Autodesk Fusion 360 part; units mm, degrees
(part 5 of 5)
  spline S1328 degree 3 poles (-71.2858, -117.1443) (-71.9506, -117.9779) (-71.7606, -118.0412) (-71.0536, -117.2287) knots 0 0 0 0 1 1 1 1
  spline S1329 degree 3 poles (-71.0536, -117.2287) (-70.7054, -116.8172) (-70.3889, -116.4795) (-70.3678, -116.4795) knots 0 0 0 0 1 1 1 1
  spline S1330 degree 3 poles (-70.3678, -116.4795) (-70.3467, -116.4795) (-70.3678, -116.5956) (-70.4205, -116.7222) knots 0 0 0 0 1 1 1 1
  spline S1331 degree 3 poles (-70.4205, -116.7222) (-70.5577, -117.0704) (-70.5682, -119.7401) (-70.4416, -120.8692) knots 0 0 0 0 1 1 1 1
  spline S1332 degree 3 poles (-70.4416, -120.8692) (-70.3783, -121.3862) (-70.3044, -122.3148) (-70.2622, -122.9374) knots 0 0 0 0 1 1 1 1
  spline S1333 degree 3 poles (-70.2622, -122.9374) (-70.1778, -124.3197) (-70.315, -124.7945) (-71.1381, -125.8708) knots 0 0 0 0 1 1 1 1
  spline S1334 degree 3 poles (-71.1381, -125.8708) (-71.7606, -126.6833) (-71.8978, -127.1054) (-71.328, -126.4512) knots 0 0 0 0 1 1 1 1
  spline S1335 degree 3 poles (-71.328, -126.4512) (-70.2728, -125.2271) (-69.1543, -122.8002) (-68.8061, -120.9114) knots 0 0 0 0 1 1 1 1
  spline S1336 degree 3 poles (-68.8061, -120.9114) (-68.6056, -119.8984) (-68.6161, -119.9617) (-68.7216, -119.9617) knots 0 0 0 0 1 1 1 1
  spline S1337 degree 3 poles (-68.7216, -119.9617) (-68.7638, -119.9617) (-68.8588, -120.3205) (-68.9327, -120.7636) knots 0 0 0 0 1 1 1 1
  spline S1338 degree 3 poles (-68.9327, -120.7636) (-69.0488, -121.5445) (-69.5764, -123.2434) (-69.8613, -123.7604) knots 0 0 0 0 1 1 1 1
  spline S1339 degree 3 poles (-69.8613, -123.7604) (-69.9879, -123.9926) (-69.9984, -123.9081) (-70.009, -122.9162) knots 0 0 0 0 1 1 1 1
  spline S1340 degree 3 poles (-70.009, -122.9162) (-70.0195, -122.3042) (-70.0406, -121.6606) (-70.0723, -121.4917) knots 0 0 0 0 1 1 1 1
  spline S1341 degree 3 poles (-70.0723, -121.4917) (-70.2517, -120.2888) (-70.3044, -117.6719) (-70.1778, -116.6378) knots 0 0 0 0 1 1 1 1
  spline S1342 degree 3 poles (-70.1778, -116.6378) (-70.1251, -116.1418) (-70.0617, -116.0574) (-69.2176, -115.2344) knots 0 0 0 0 1 1 1 1
  spline S1343 degree 3 poles (-69.2176, -115.2344) (-68.2468, -114.3058) (-68.1413, -114.0842) (-69.0065, -114.8123) knots 0 0 0 0 1 1 1 1
  spline S1344 degree 3 poles (-42.4787, -115.3927) (-41.7084, -116.1313) (-41.6029, -116.2685) (-41.5185, -116.7433) knots 0 0 0 0 1 1 1 1
  spline S1345 degree 3 poles (-41.5185, -116.7433) (-41.413, -117.3026) (-41.4657, -120.9219) (-41.5818, -121.5445) knots 0 0 0 0 1 1 1 1
  spline S1346 degree 3 poles (-41.5818, -121.5445) (-41.624, -121.745) (-41.6662, -122.4203) (-41.6662, -123.0429) knots 0 0 0 0 1 1 1 1
  spline S1347 degree 3 poles (-41.6662, -123.0429) (-41.6768, -123.6654) (-41.7084, -124.1403) (-41.7401, -124.0981) knots 0 0 0 0 1 1 1 1
  spline S1348 degree 3 poles (-41.7401, -124.0981) (-41.93, -123.8976) (-42.5948, -121.861) (-42.7531, -120.9958) knots 0 0 0 0 1 1 1 1
  spline S1349 degree 3 poles (-42.7531, -120.9958) (-42.8586, -120.4576) (-42.9536, -120.12) (-42.9747, -120.2466) knots 0 0 0 0 1 1 1 1
  spline S1350 degree 3 poles (-42.9747, -120.2466) (-43.0802, -120.9747) (-42.3416, -123.3489) (-41.5502, -124.8051) knots 0 0 0 0 1 1 1 1
  spline S1351 degree 3 poles (-41.5502, -124.8051) (-41.0226, -125.8075) (-40.1256, -127.0104) (-40.0623, -126.8311) knots 0 0 0 0 1 1 1 1
  spline S1352 degree 3 poles (-40.0623, -126.8311) (-40.0412, -126.7572) (-40.1573, -126.5356) (-40.3261, -126.314) knots 0 0 0 0 1 1 1 1
  spline S1353 degree 3 poles (-40.3261, -126.314) (-40.6427, -125.8919) (-40.8326, -125.5859) (-41.2653, -124.7734) knots 0 0 0 0 1 1 1 1
  spline S1354 degree 3 poles (-41.2653, -124.7734) (-41.5185, -124.288) (-41.5291, -124.2036) (-41.4763, -123.1378) knots 0 0 0 0 1 1 1 1
  spline S1355 degree 3 poles (-41.4763, -123.1378) (-41.4446, -122.5258) (-41.3813, -121.6606) (-41.3391, -121.2279) knots 0 0 0 0 1 1 1 1
  spline S1356 degree 3 poles (-41.3391, -121.2279) (-41.2864, -120.7953) (-41.2547, -119.5924) (-41.2547, -118.5688) knots 0 0 0 0 1 1 1 1
  line L192 (-41.2547, -118.5688) -> (-41.2547, -116.7011)
  line L193 (-41.2547, -116.7011) -> (-40.9487, -116.986)
  spline S1357 degree 3 poles (-40.9487, -116.986) (-40.7799, -117.1443) (-40.5161, -117.4609) (-40.3472, -117.6824) knots 0 0 0 0 1 1 1 1
  spline S1358 degree 3 poles (-40.3472, -117.6824) (-40.1784, -117.904) (-40.0412, -118.0201) (-40.0412, -117.9357) knots 0 0 0 0 1 1 1 1
  spline S1359 degree 3 poles (-40.0412, -117.9357) (-40.0412, -117.6297) (-41.1386, -116.3845) (-42.4154, -115.2449) knots 0 0 0 0 1 1 1 1
  spline S1360 degree 3 poles (-42.4154, -115.2449) (-43.4601, -114.3058) (-43.5128, -114.4219) (-42.4787, -115.3927) knots 0 0 0 0 1 1 1 1
  spline S1361 degree 3 poles (-65.039, -118.3367) (-65.039, -118.4527) (-65.0073, -118.4844) (-64.9757, -118.4) knots 0 0 0 0 1 1 1 1
  spline S1362 degree 3 poles (-64.9757, -118.4) (-64.944, -118.3261) (-64.9546, -118.2311) (-64.9862, -118.1995) knots 0 0 0 0 1 1 1 1
  spline S1363 degree 3 poles (-64.9862, -118.1995) (-65.0179, -118.1573) (-65.0495, -118.2206) (-65.039, -118.3367) knots 0 0 0 0 1 1 1 1
  spline S1364 degree 3 poles (-68.7111, -119.3813) (-68.7111, -119.6135) (-68.69, -119.6979) (-68.6689, -119.5607) knots 0 0 0 0 1 1 1 1
  spline S1365 degree 3 poles (-68.6689, -119.5607) (-68.6478, -119.4341) (-68.6478, -119.2441) (-68.6689, -119.1386) knots 0 0 0 0 1 1 1 1
  spline S1366 degree 3 poles (-68.6689, -119.1386) (-68.7005, -119.0437) (-68.7216, -119.1492) (-68.7111, -119.3813) knots 0 0 0 0 1 1 1 1
  spline S1367 degree 3 poles (-46.7734, -119.4868) (-46.6785, -119.7084) (-46.6996, -119.8034) (-46.9528, -120.1411) knots 0 0 0 0 1 1 1 1
  spline S1368 degree 3 poles (-46.9528, -120.1411) (-47.1111, -120.3627) (-47.4382, -120.7425) (-47.6809, -120.9852) knots 0 0 0 0 1 1 1 1
  spline S1369 degree 3 poles (-47.6809, -120.9852) (-47.913, -121.2385) (-48.0502, -121.439) (-47.9869, -121.439) knots 0 0 0 0 1 1 1 1
  spline S1370 degree 3 poles (-47.9869, -121.439) (-47.8497, -121.439) (-47.1005, -120.6159) (-46.7207, -120.0461) knots 0 0 0 0 1 1 1 1
  spline S1371 degree 3 poles (-46.7207, -120.0461) (-46.4991, -119.719) (-46.478, -119.6346) (-46.6046, -119.4446) knots 0 0 0 0 1 1 1 1
  spline S1372 degree 3 poles (-46.6046, -119.4446) (-46.7945, -119.1386) (-46.9211, -119.1703) (-46.7734, -119.4868) knots 0 0 0 0 1 1 1 1
  spline S1373 degree 3 poles (-42.7003, -119.5396) (-42.8586, -119.7401) (-42.9641, -119.9195) (-42.9325, -119.9511) knots 0 0 0 0 1 1 1 1
  spline S1374 degree 3 poles (-42.9325, -119.9511) (-42.9114, -119.9722) (-42.827, -119.9089) (-42.7425, -119.8034) knots 0 0 0 0 1 1 1 1
  spline S1375 degree 3 poles (-42.7425, -119.8034) (-42.6265, -119.6346) (-42.5948, -119.7506) (-42.5315, -120.6581) knots 0 0 0 0 1 1 1 1
  spline S1376 degree 3 poles (-42.5315, -120.6581) (-42.426, -122.2937) (-42.2994, -122.4731) (-42.331, -120.9536) knots 0 0 0 0 1 1 1 1
  spline S1377 degree 3 poles (-42.331, -120.9536) (-42.3838, -119.012) (-42.3627, -119.107) (-42.7003, -119.5396) knots 0 0 0 0 1 1 1 1
  spline S1378 degree 3 poles (-48.8416, -122.4414) (-48.9366, -122.7158) (-48.9155, -122.7791) (-48.7889, -122.568) knots 0 0 0 0 1 1 1 1
  spline S1379 degree 3 poles (-48.7889, -122.568) (-48.7255, -122.4625) (-48.6939, -122.3464) (-48.7255, -122.3253) knots 0 0 0 0 1 1 1 1
  spline S1380 degree 3 poles (-48.7255, -122.3253) (-48.7466, -122.2937) (-48.7994, -122.3464) (-48.8416, -122.4414) knots 0 0 0 0 1 1 1 1
  spline S1381 degree 3 poles (-62.9391, -123.1273) (-62.9391, -123.1801) (-62.8864, -123.2328) (-62.8336, -123.2328) knots 0 0 0 0 1 1 1 1
  spline S1382 degree 3 poles (-62.8336, -123.2328) (-62.7703, -123.2328) (-62.7281, -123.1801) (-62.7281, -123.1273) knots 0 0 0 0 1 1 1 1
  spline S1383 degree 3 poles (-62.7281, -123.1273) (-62.7281, -123.064) (-62.7703, -123.0218) (-62.8336, -123.0218) knots 0 0 0 0 1 1 1 1
  spline S1384 degree 3 poles (-62.8336, -123.0218) (-62.8864, -123.0218) (-62.9391, -123.064) (-62.9391, -123.1273) knots 0 0 0 0 1 1 1 1
  spline S1385 degree 3 poles (-69.6397, -125.1955) (-70.0829, -125.8708) (-70.8954, -126.7044) (-71.3808, -126.9893) knots 0 0 0 0 1 1 1 1
  spline S1386 degree 3 poles (-71.3808, -126.9893) (-71.6657, -127.1582) (-71.8028, -127.3481) (-71.634, -127.3481) knots 0 0 0 0 1 1 1 1
  spline S1387 degree 3 poles (-71.634, -127.3481) (-71.5285, -127.3481) (-70.927, -126.9155) (-70.5577, -126.5673) knots 0 0 0 0 1 1 1 1
  spline S1388 degree 3 poles (-70.5577, -126.5673) (-70.3783, -126.3984) (-70.22, -126.2823) (-70.22, -126.3351) knots 0 0 0 0 1 1 1 1
  spline S1389 degree 3 poles (-70.22, -126.3351) (-70.22, -126.4617) (-71.0325, -127.8018) (-71.3702, -128.2345) knots 0 0 0 0 1 1 1 1
  spline S1390 degree 3 poles (-71.3702, -128.2345) (-71.5496, -128.4561) (-71.6973, -128.7093) (-71.6973, -128.8043) knots 0 0 0 0 1 1 1 1
  spline S1391 degree 3 poles (-71.6973, -128.8043) (-71.6973, -128.9942) (-71.6762, -128.9731) (-71.2014, -128.3505) knots 0 0 0 0 1 1 1 1
  spline S1392 degree 3 poles (-71.2014, -128.3505) (-70.7371, -127.7491) (-70.1778, -126.7677) (-69.8507, -125.9763) knots 0 0 0 0 1 1 1 1
  spline S1393 degree 3 poles (-69.8507, -125.9763) (-69.6924, -125.5965) (-69.4708, -125.1533) (-69.3548, -124.995) knots 0 0 0 0 1 1 1 1
  spline S1394 degree 3 poles (-69.3548, -124.995) (-69.2387, -124.8262) (-69.1648, -124.6784) (-69.1859, -124.6468) knots 0 0 0 0 1 1 1 1
  spline S1395 degree 3 poles (-69.1859, -124.6468) (-69.2176, -124.6257) (-69.4181, -124.8684) (-69.6397, -125.1955) knots 0 0 0 0 1 1 1 1
  spline S1396 degree 3 poles (-42.4682, -124.9211) (-42.4682, -124.9739) (-42.4154, -125.0267) (-42.3521, -125.0267) knots 0 0 0 0 1 1 1 1
  spline S1397 degree 3 poles (-42.3521, -125.0267) (-42.2994, -125.0267) (-42.2783, -124.9739) (-42.3099, -124.9211) knots 0 0 0 0 1 1 1 1
  spline S1398 degree 3 poles (-42.3099, -124.9211) (-42.3416, -124.8578) (-42.3943, -124.8156) (-42.426, -124.8156) knots 0 0 0 0 1 1 1 1
  spline S1399 degree 3 poles (-42.426, -124.8156) (-42.4471, -124.8156) (-42.4682, -124.8578) (-42.4682, -124.9211) knots 0 0 0 0 1 1 1 1
  spline S1400 degree 3 poles (-42.2149, -125.4171) (-42.1305, -125.5859) (-41.8351, -126.1557) (-41.5713, -126.6939) knots 0 0 0 0 1 1 1 1
  spline S1401 degree 3 poles (-41.5713, -126.6939) (-41.0964, -127.6647) (-40.3578, -128.857) (-40.1467, -128.9837) knots 0 0 0 0 1 1 1 1
  spline S1402 degree 3 poles (-40.1467, -128.9837) (-39.9463, -129.1103) (-40.0412, -128.9098) (-40.5055, -128.2028) knots 0 0 0 0 1 1 1 1
  spline S1403 degree 3 poles (-40.5055, -128.2028) (-41.2442, -127.0737) (-41.5924, -126.4195) (-41.3497, -126.62) knots 0 0 0 0 1 1 1 1
  spline S1404 degree 3 poles (-41.3497, -126.62) (-41.2442, -126.7044) (-40.8959, -126.9788) (-40.5899, -127.232) knots 0 0 0 0 1 1 1 1
  spline S1405 degree 3 poles (-40.5899, -127.232) (-40.2628, -127.5064) (-40.0412, -127.6225) (-40.0412, -127.538) knots 0 0 0 0 1 1 1 1
  spline S1406 degree 3 poles (-40.0412, -127.538) (-40.0412, -127.4536) (-40.2523, -127.2426) (-40.5055, -127.0632) knots 0 0 0 0 1 1 1 1
  spline S1407 degree 3 poles (-40.5055, -127.0632) (-40.9487, -126.7466) (-42.1516, -125.396) (-42.1516, -125.2166) knots 0 0 0 0 1 1 1 1
  spline S1408 degree 3 poles (-42.1516, -125.2166) (-42.1516, -125.1744) (-42.2044, -125.1322) (-42.2677, -125.1322) knots 0 0 0 0 1 1 1 1
  spline S1409 degree 3 poles (-42.2677, -125.1322) (-42.331, -125.1322) (-42.3099, -125.2482) (-42.2149, -125.4171) knots 0 0 0 0 1 1 1 1
  spline S1410 degree 3 poles (-51.8595, -127.2848) (-51.8595, -127.3059) (-51.7856, -127.3587) (-51.6907, -127.3903) knots 0 0 0 0 1 1 1 1
  spline S1411 degree 3 poles (-51.6907, -127.3903) (-51.6062, -127.422) (-51.564, -127.4114) (-51.5957, -127.3481) knots 0 0 0 0 1 1 1 1
  spline S1412 degree 3 poles (-51.5957, -127.3481) (-51.659, -127.2426) (-51.8595, -127.2004) (-51.8595, -127.2848) knots 0 0 0 0 1 1 1 1
  spline S1413 degree 3 poles (-46.4252, -132.2653) (-46.594, -132.3603) (-46.9211, -132.5291) (-47.1427, -132.6452) knots 0 0 0 0 1 1 1 1
  spline S1414 degree 3 poles (-47.1427, -132.6452) (-47.3749, -132.7507) (-47.5332, -132.8774) (-47.5015, -132.8985) knots 0 0 0 0 1 1 1 1
  spline S1415 degree 3 poles (-47.5015, -132.8985) (-47.4487, -132.9618) (-45.9504, -132.2337) (-45.9504, -132.1493) knots 0 0 0 0 1 1 1 1
  spline S1416 degree 3 poles (-45.9504, -132.1493) (-45.9504, -132.0543) (-46.0981, -132.0965) (-46.4252, -132.2653) knots 0 0 0 0 1 1 1 1
  spline S1417 degree 3 poles (-71.6973, -132.5608) (-71.6973, -132.7296) (-71.4335, -132.9723) (-70.9587, -133.2045) knots 0 0 0 0 1 1 1 1
  spline S1418 degree 3 poles (-70.9587, -133.2045) (-70.7582, -133.31) (-70.6527, -133.4155) (-70.7265, -133.4366) knots 0 0 0 0 1 1 1 1
  spline S1419 degree 3 poles (-70.7265, -133.4366) (-70.9587, -133.521) (-70.8637, -133.6899) (-70.4838, -133.8482) knots 0 0 0 0 1 1 1 1
  spline S1420 degree 3 poles (-70.4838, -133.8482) (-70.0512, -134.0275) (-70.009, -134.1542) (-70.3678, -134.2491) knots 0 0 0 0 1 1 1 1
  spline S1421 degree 3 poles (-70.3678, -134.2491) (-70.6632, -134.323) (-71.3069, -134.9245) (-71.2225, -135.0511) knots 0 0 0 0 1 1 1 1
  spline S1422 degree 3 poles (-71.2225, -135.0511) (-71.1908, -135.0933) (-71.0114, -135.1355) (-70.8109, -135.1355) knots 0 0 0 0 1 1 1 1
  spline S1423 degree 3 poles (-70.8109, -135.1355) (-70.3783, -135.1355) (-69.703, -135.5576) (-69.7768, -135.7897) knots 0 0 0 0 1 1 1 1
  spline S1424 degree 3 poles (-69.7768, -135.7897) (-69.8085, -135.8741) (-69.6608, -135.8003) (-69.4497, -135.6314) knots 0 0 0 0 1 1 1 1
  spline S1425 degree 3 poles (-69.4497, -135.6314) (-69.0171, -135.2621) (-68.9327, -135.0511) (-69.3337, -135.3149) knots 0 0 0 0 1 1 1 1
  spline S1426 degree 3 poles (-69.3337, -135.3149) (-69.5764, -135.4732) (-69.6186, -135.4732) (-69.8613, -135.3149) knots 0 0 0 0 1 1 1 1
  spline S1427 degree 3 poles (-69.8613, -135.3149) (-70.1673, -135.1144) (-70.1884, -135.0511) (-69.9035, -135.1249) knots 0 0 0 0 1 1 1 1
  spline S1428 degree 3 poles (-69.9035, -135.1249) (-69.7874, -135.1566) (-69.6924, -135.1249) (-69.6924, -135.0616) knots 0 0 0 0 1 1 1 1
  spline S1429 degree 3 poles (-69.6924, -135.0616) (-69.6924, -134.935) (-70.0406, -134.8928) (-70.6421, -134.935) knots 0 0 0 0 1 1 1 1
  line L194 (-70.6421, -134.935) -> (-71.0114, -134.9561)
  line L195 (-71.0114, -134.9561) -> (-70.7582, -134.6923)
  spline S1430 degree 3 poles (-70.7582, -134.6923) (-70.5999, -134.5235) (-70.3255, -134.3863) (-70.0934, -134.3546) knots 0 0 0 0 1 1 1 1
  spline S1431 degree 3 poles (-70.0934, -134.3546) (-69.6713, -134.2808) (-69.5764, -134.1647) (-69.8507, -134.0592) knots 0 0 0 0 1 1 1 1
  spline S1432 degree 3 poles (-69.8507, -134.0592) (-70.009, -134.0064) (-70.0829, -133.7637) (-69.9246, -133.8059) knots 0 0 0 0 1 1 1 1
  spline S1433 degree 3 poles (-69.9246, -133.8059) (-69.7874, -133.8482) (-69.3759, -133.6688) (-69.3759, -133.5738) knots 0 0 0 0 1 1 1 1
  spline S1434 degree 3 poles (-69.3759, -133.5738) (-69.3759, -133.5105) (-69.4919, -133.521) (-69.6502, -133.5738) knots 0 0 0 0 1 1 1 1
  spline S1435 degree 3 poles (-69.6502, -133.5738) (-70.1778, -133.7743) (-70.8109, -133.6477) (-70.4311, -133.4155) knots 0 0 0 0 1 1 1 1
  spline S1436 degree 3 poles (-70.4311, -133.4155) (-70.2306, -133.2889) (-70.3255, -133.1834) (-70.7265, -133.0673) knots 0 0 0 0 1 1 1 1
  spline S1437 degree 3 poles (-70.7265, -133.0673) (-70.9587, -132.9934) (-71.2647, -132.8246) (-71.4124, -132.6874) knots 0 0 0 0 1 1 1 1
  spline S1438 degree 3 poles (-71.4124, -132.6874) (-71.5812, -132.5291) (-71.6973, -132.4764) (-71.6973, -132.5608) knots 0 0 0 0 1 1 1 1
  spline S1439 degree 3 poles (-64.0049, -133.2572) (-63.6356, -133.5316) (-63.0974, -134.1858) (-63.1818, -134.2702) knots 0 0 0 0 1 1 1 1
  spline S1440 degree 3 poles (-63.1818, -134.2702) (-63.1924, -134.2913) (-63.4667, -134.2069) (-63.7833, -134.1014) knots 0 0 0 0 1 1 1 1
  spline S1441 degree 3 poles (-63.7833, -134.1014) (-64.3848, -133.8904) (-65.3133, -133.827) (-65.556, -133.9748) knots 0 0 0 0 1 1 1 1
  spline S1442 degree 3 poles (-65.556, -133.9748) (-65.6404, -134.0381) (-65.556, -134.1331) (-65.2606, -134.3019) knots 0 0 0 0 1 1 1 1
  spline S1443 degree 3 poles (-65.2606, -134.3019) (-65.0284, -134.4285) (-64.8385, -134.4918) (-64.8385, -134.4391) knots 0 0 0 0 1 1 1 1
  spline S1444 degree 3 poles (-64.8385, -134.4391) (-64.8385, -134.3758) (-64.9124, -134.3124) (-64.9968, -134.2702) knots 0 0 0 0 1 1 1 1
  spline S1445 degree 3 poles (-64.9968, -134.2702) (-65.0812, -134.2386) (-65.1551, -134.1647) (-65.1551, -134.1014) knots 0 0 0 0 1 1 1 1
  spline S1446 degree 3 poles (-65.1551, -134.1014) (-65.1551, -133.9853) (-64.8068, -134.0275) (-63.8466, -134.2702) knots 0 0 0 0 1 1 1 1
  spline S1447 degree 3 poles (-63.8466, -134.2702) (-63.4456, -134.3652) (-63.1818, -134.3863) (-63.1185, -134.323) knots 0 0 0 0 1 1 1 1
  spline S1448 degree 3 poles (-63.1185, -134.323) (-62.9075, -134.112) (-63.8888, -132.9407) (-64.2792, -132.9407) knots 0 0 0 0 1 1 1 1
  spline S1449 degree 3 poles (-64.2792, -132.9407) (-64.3742, -132.9407) (-64.2476, -133.0884) (-64.0049, -133.2572) knots 0 0 0 0 1 1 1 1
  spline S1450 degree 3 poles (-60.1956, -133.1412) (-60.1956, -133.1939) (-60.0795, -133.31) (-59.9318, -133.405) knots 0 0 0 0 1 1 1 1
  spline S1451 degree 3 poles (-59.9318, -133.405) (-59.7841, -133.4999) (-59.668, -133.5316) (-59.668, -133.4788) knots 0 0 0 0 1 1 1 1
  spline S1452 degree 3 poles (-59.668, -133.4788) (-59.668, -133.4261) (-59.7841, -133.31) (-59.9318, -133.215) knots 0 0 0 0 1 1 1 1
  spline S1453 degree 3 poles (-59.9318, -133.215) (-60.0795, -133.1201) (-60.1956, -133.0884) (-60.1956, -133.1412) knots 0 0 0 0 1 1 1 1
  spline S1454 degree 3 poles (-40.5477, -133.215) (-40.8432, -133.3417) (-40.8854, -133.3944) (-40.7693, -133.5316) knots 0 0 0 0 1 1 1 1
  spline S1455 degree 3 poles (-40.7693, -133.5316) (-40.706, -133.616) (-40.6638, -133.711) (-40.6955, -133.7321) knots 0 0 0 0 1 1 1 1
  spline S1456 degree 3 poles (-40.6955, -133.7321) (-40.7799, -133.8165) (-41.2442, -133.8165) (-41.5607, -133.7321) knots 0 0 0 0 1 1 1 1
  spline S1457 degree 3 poles (-41.5607, -133.7321) (-41.7718, -133.6793) (-41.8456, -133.6793) (-41.7929, -133.7637) knots 0 0 0 0 1 1 1 1
  spline S1458 degree 3 poles (-41.7929, -133.7637) (-41.7612, -133.827) (-41.5713, -133.9115) (-41.3919, -133.9431) knots 0 0 0 0 1 1 1 1
  line L196 (-41.3919, -133.9431) -> (-41.0542, -134.017)
  line L197 (-41.0542, -134.017) -> (-41.2864, -134.2069)
  line L198 (-41.2864, -134.2069) -> (-41.508, -134.3969)
  line L199 (-41.508, -134.3969) -> (-41.1281, -134.4496)
  spline S1459 degree 3 poles (-41.1281, -134.4496) (-40.7904, -134.5129) (-40.2523, -134.8717) (-40.2523, -135.0511) knots 0 0 0 0 1 1 1 1
  spline S1460 degree 3 poles (-40.2523, -135.0511) (-40.2523, -135.0827) (-40.4211, -135.0933) (-40.6216, -135.0722) knots 0 0 0 0 1 1 1 1
  spline S1461 degree 3 poles (-40.6216, -135.0722) (-40.8221, -135.0511) (-41.1175, -135.0616) (-41.2758, -135.1038) knots 0 0 0 0 1 1 1 1
  line L200 (-41.2758, -135.1038) -> (-41.5713, -135.1883)
  line L201 (-41.5713, -135.1883) -> (-41.3075, -135.2621)
  line L202 (-41.3075, -135.2621) -> (-41.0437, -135.3254)
  line L203 (-41.0437, -135.3254) -> (-41.3708, -135.5048)
  spline S1462 degree 3 poles (-41.3708, -135.5048) (-41.6662, -135.6525) (-41.719, -135.6631) (-41.8351, -135.5259) knots 0 0 0 0 1 1 1 1
  spline S1463 degree 3 poles (-41.8351, -135.5259) (-41.9089, -135.4415) (-42.0145, -135.3676) (-42.0778, -135.3676) knots 0 0 0 0 1 1 1 1
  spline S1464 degree 3 poles (-42.0778, -135.3676) (-42.1305, -135.3676) (-42.0989, -135.4626) (-41.9933, -135.5787) knots 0 0 0 0 1 1 1 1
  spline S1465 degree 3 poles (-41.9933, -135.5787) (-41.7401, -135.8636) (-41.3919, -135.8425) (-41.0964, -135.5259) knots 0 0 0 0 1 1 1 1
  spline S1466 degree 3 poles (-41.0964, -135.5259) (-40.917, -135.336) (-40.7377, -135.2621) (-40.4422, -135.2621) knots 0 0 0 0 1 1 1 1
  spline S1467 degree 3 poles (-40.4422, -135.2621) (-40.2206, -135.2621) (-40.0412, -135.2199) (-40.0412, -135.1672) knots 0 0 0 0 1 1 1 1
  spline S1468 degree 3 poles (-40.0412, -135.1672) (-40.0412, -134.935) (-40.5477, -134.3652) (-40.8115, -134.3124) knots 0 0 0 0 1 1 1 1
  spline S1469 degree 3 poles (-40.8115, -134.3124) (-41.1492, -134.2491) (-41.0648, -134.0908) (-40.5899, -133.9009) knots 0 0 0 0 1 1 1 1
  spline S1470 degree 3 poles (-40.5899, -133.9009) (-40.2417, -133.7532) (-40.1362, -133.5738) (-40.4105, -133.5738) knots 0 0 0 0 1 1 1 1
  spline S1471 degree 3 poles (-40.4105, -133.5738) (-40.6532, -133.5738) (-40.6005, -133.3839) (-40.3367, -133.3417) knots 0 0 0 0 1 1 1 1
  spline S1472 degree 3 poles (-40.3367, -133.3417) (-40.2101, -133.3206) (-40.094, -133.2467) (-40.0623, -133.1728) knots 0 0 0 0 1 1 1 1
  spline S1473 degree 3 poles (-40.0623, -133.1728) (-40.0096, -133.0145) (-40.1045, -133.0251) (-40.5477, -133.215) knots 0 0 0 0 1 1 1 1
  spline S1474 degree 3 poles (-65.4716, -133.2572) (-65.4716, -133.31) (-65.4083, -133.3628) (-65.3239, -133.3628) knots 0 0 0 0 1 1 1 1
  spline S1475 degree 3 poles (-65.3239, -133.3628) (-65.25, -133.3628) (-65.1234, -133.4366) (-65.0495, -133.521) knots 0 0 0 0 1 1 1 1
  spline S1476 degree 3 poles (-65.0495, -133.521) (-64.9124, -133.6899) (-64.733, -133.7321) (-64.733, -133.5949) knots 0 0 0 0 1 1 1 1
  spline S1477 degree 3 poles (-64.733, -133.5949) (-64.733, -133.5105) (-65.2817, -133.1517) (-65.4083, -133.1517) knots 0 0 0 0 1 1 1 1
  spline S1478 degree 3 poles (-65.4083, -133.1517) (-65.44, -133.1517) (-65.4716, -133.1939) (-65.4716, -133.2572) knots 0 0 0 0 1 1 1 1
  spline S1479 degree 3 poles (-65.3344, -133.6477) (-65.2395, -133.7426) (-65.1234, -133.7848) (-65.0812, -133.7426) knots 0 0 0 0 1 1 1 1
  spline S1480 degree 3 poles (-65.0812, -133.7426) (-65.039, -133.7004) (-65.0706, -133.6266) (-65.1551, -133.5738) knots 0 0 0 0 1 1 1 1
  spline S1481 degree 3 poles (-65.1551, -133.5738) (-65.4189, -133.405) (-65.5244, -133.4577) (-65.3344, -133.6477) knots 0 0 0 0 1 1 1 1
  spline S1482 degree 3 poles (-45.8448, -133.5738) (-45.9715, -133.6582) (-45.9609, -133.6793) (-45.771, -133.6793) knots 0 0 0 0 1 1 1 1
  spline S1483 degree 3 poles (-45.771, -133.6793) (-45.6444, -133.6793) (-45.5072, -133.6266) (-45.4755, -133.5738) knots 0 0 0 0 1 1 1 1
  spline S1484 degree 3 poles (-45.4755, -133.5738) (-45.3911, -133.4366) (-45.6338, -133.4366) (-45.8448, -133.5738) knots 0 0 0 0 1 1 1 1
  spline S1485 degree 3 poles (-46.4358, -133.7321) (-46.5413, -133.8165) (-46.5835, -133.8904) (-46.5096, -133.8904) knots 0 0 0 0 1 1 1 1
  spline S1486 degree 3 poles (-46.5096, -133.8904) (-46.3091, -133.8904) (-46.0559, -133.7743) (-46.0559, -133.6688) knots 0 0 0 0 1 1 1 1
  spline S1487 degree 3 poles (-46.0559, -133.6688) (-46.0559, -133.5316) (-46.2036, -133.5527) (-46.4358, -133.7321) knots 0 0 0 0 1 1 1 1
  spline S1488 degree 3 poles (-46.9423, -134.1964) (-47.2483, -134.534) (-47.0689, -134.6818) (-46.3935, -134.6501) knots 0 0 0 0 1 1 1 1
  spline S1489 degree 3 poles (-46.3935, -134.6501) (-45.8132, -134.6185) (-45.771, -134.629) (-45.7815, -134.8506) knots 0 0 0 0 1 1 1 1
  spline S1490 degree 3 poles (-45.7815, -134.8506) (-45.7921, -135.0089) (-45.7182, -135.0933) (-45.5494, -135.1144) knots 0 0 0 0 1 1 1 1
  spline S1491 degree 3 poles (-45.5494, -135.1144) (-45.4122, -135.1355) (-45.159, -135.241) (-44.969, -135.3465) knots 0 0 0 0 1 1 1 1
  spline S1492 degree 3 poles (-44.969, -135.3465) (-44.6419, -135.5259) (-44.6841, -135.5259) (-47.1111, -135.5576) knots 0 0 0 0 1 1 1 1
  spline S1493 degree 3 poles (-47.1111, -135.5576) (-48.5462, -135.5681) (-49.6225, -135.6209) (-49.6858, -135.6842) knots 0 0 0 0 1 1 1 1
  spline S1494 degree 3 poles (-49.6858, -135.6842) (-49.7596, -135.7581) (-48.81, -135.7897) (-46.9528, -135.7897) knots 0 0 0 0 1 1 1 1
  spline S1495 degree 3 poles (-46.9528, -135.7897) (-44.1671, -135.7897) (-44.1249, -135.7897) (-44.3042, -135.5892) knots 0 0 0 0 1 1 1 1
  spline S1496 degree 3 poles (-44.3042, -135.5892) (-44.4098, -135.4732) (-44.663, -135.2938) (-44.8741, -135.1988) knots 0 0 0 0 1 1 1 1
  spline S1497 degree 3 poles (-44.8741, -135.1988) (-45.2961, -134.9983) (-45.3278, -134.9878) (-45.6021, -134.9561) knots 0 0 0 0 1 1 1 1
  spline S1498 degree 3 poles (-45.6021, -134.9561) (-45.7499, -134.935) (-45.7288, -134.9034) (-45.5283, -134.8295) knots 0 0 0 0 1 1 1 1
  spline S1499 degree 3 poles (-45.5283, -134.8295) (-45.3806, -134.7662) (-45.0956, -134.7451) (-44.8952, -134.7767) knots 0 0 0 0 1 1 1 1
  line L204 (-44.8952, -134.7767) -> (-44.5258, -134.8295)
  line L205 (-44.5258, -134.8295) -> (-44.8424, -134.6501)
  spline S1500 degree 3 poles (-44.8424, -134.6501) (-45.064, -134.5235) (-45.4228, -134.4813) (-46.077, -134.4707) knots 0 0 0 0 1 1 1 1
  line L206 (-46.077, -134.4707) -> (-46.995, -134.4707)
  line L207 (-46.995, -134.4707) -> (-46.7734, -134.228)
  spline S1501 degree 3 poles (-46.7734, -134.228) (-46.6468, -134.1014) (-46.594, -133.9959) (-46.6573, -133.9959) knots 0 0 0 0 1 1 1 1
  spline S1502 degree 3 poles (-46.6573, -133.9959) (-46.7101, -133.9959) (-46.8367, -134.0803) (-46.9423, -134.1964) knots 0 0 0 0 1 1 1 1
  spline S1503 degree 3 poles (-65.6827, -134.7978) (-65.8831, -134.8823) (-66.0731, -134.9878) (-66.1047, -135.03) knots 0 0 0 0 1 1 1 1
  spline S1504 degree 3 poles (-66.1047, -135.03) (-66.1364, -135.0722) (-66.358, -135.241) (-66.6007, -135.4099) knots 0 0 0 0 1 1 1 1
  spline S1505 degree 3 poles (-66.6007, -135.4099) (-66.8539, -135.5787) (-67.0544, -135.7264) (-67.0544, -135.7475) knots 0 0 0 0 1 1 1 1
  spline S1506 degree 3 poles (-67.0544, -135.7475) (-67.0544, -135.7686) (-65.746, -135.7897) (-64.1421, -135.7897) knots 0 0 0 0 1 1 1 1
  spline S1507 degree 3 poles (-64.1421, -135.7897) (-62.2321, -135.7897) (-61.2614, -135.7581) (-61.3036, -135.6842) knots 0 0 0 0 1 1 1 1
  spline S1508 degree 3 poles (-61.3036, -135.6842) (-61.3458, -135.6209) (-62.306, -135.5787) (-63.8466, -135.5787) knots 0 0 0 0 1 1 1 1
  spline S1509 degree 3 poles (-63.8466, -135.5787) (-65.2078, -135.5787) (-66.3158, -135.5365) (-66.3158, -135.4837) knots 0 0 0 0 1 1 1 1
  spline S1510 degree 3 poles (-66.3158, -135.4837) (-66.3158, -135.3887) (-66.0942, -135.1672) (-65.9992, -135.1777) knots 0 0 0 0 1 1 1 1
  spline S1511 degree 3 poles (-65.9992, -135.1777) (-65.9676, -135.1883) (-65.7038, -135.0616) (-65.4189, -134.9139) knots 0 0 0 0 1 1 1 1
  spline S1512 degree 3 poles (-65.4189, -134.9139) (-64.849, -134.6185) (-65.0495, -134.5235) (-65.6827, -134.7978) knots 0 0 0 0 1 1 1 1
  spline S1513 degree 3 poles (-59.5625, -134.9456) (-59.5625, -134.9983) (-59.4886, -135.0194) (-59.4042, -134.9878) knots 0 0 0 0 1 1 1 1
  spline S1514 degree 3 poles (-59.4042, -134.9878) (-59.3198, -134.9456) (-59.2459, -134.9034) (-59.2459, -134.8823) knots 0 0 0 0 1 1 1 1
  spline S1515 degree 3 poles (-59.2459, -134.8823) (-59.2459, -134.8611) (-59.3198, -134.84) (-59.4042, -134.84) knots 0 0 0 0 1 1 1 1
  spline S1516 degree 3 poles (-59.4042, -134.84) (-59.4886, -134.84) (-59.5625, -134.8823) (-59.5625, -134.9456) knots 0 0 0 0 1 1 1 1
  spline S1517 degree 3 poles (-59.5097, -135.6842) (-59.5414, -135.737) (-59.4992, -135.7897) (-59.4042, -135.7897) knots 0 0 0 0 1 1 1 1
  spline S1518 degree 3 poles (-59.4042, -135.7897) (-59.3092, -135.7897) (-59.267, -135.737) (-59.2987, -135.6842) knots 0 0 0 0 1 1 1 1
  spline S1519 degree 3 poles (-59.2987, -135.6842) (-59.3303, -135.6209) (-59.3831, -135.5787) (-59.4042, -135.5787) knots 0 0 0 0 1 1 1 1
  spline S1520 degree 3 poles (-59.4042, -135.5787) (-59.4253, -135.5787) (-59.4781, -135.6209) (-59.5097, -135.6842) knots 0 0 0 0 1 1 1 1
  spline S1521 degree 3 poles (-52.8619, -135.6842) (-52.8936, -135.737) (-52.8514, -135.7897) (-52.7564, -135.7897) knots 0 0 0 0 1 1 1 1
  spline S1522 degree 3 poles (-52.7564, -135.7897) (-52.6615, -135.7897) (-52.6192, -135.737) (-52.6509, -135.6842) knots 0 0 0 0 1 1 1 1
  spline S1523 degree 3 poles (-52.6509, -135.6842) (-52.6826, -135.6209) (-52.7353, -135.5787) (-52.7564, -135.5787) knots 0 0 0 0 1 1 1 1
  spline S1524 degree 3 poles (-52.7564, -135.5787) (-52.7775, -135.5787) (-52.8303, -135.6209) (-52.8619, -135.6842) knots 0 0 0 0 1 1 1 1
  spline S1525 degree 3 poles (-51.5957, -135.6842) (-51.6274, -135.737) (-51.6062, -135.7897) (-51.5535, -135.7897) knots 0 0 0 0 1 1 1 1
  spline S1526 degree 3 poles (-51.5535, -135.7897) (-51.4902, -135.7897) (-51.4374, -135.737) (-51.4374, -135.6842) knots 0 0 0 0 1 1 1 1
  spline S1527 degree 3 poles (-51.4374, -135.6842) (-51.4374, -135.6209) (-51.4585, -135.5787) (-51.4796, -135.5787) knots 0 0 0 0 1 1 1 1
  spline S1528 degree 3 poles (-51.4796, -135.5787) (-51.5113, -135.5787) (-51.564, -135.6209) (-51.5957, -135.6842) knots 0 0 0 0 1 1 1 1
  spline S1529 degree 3 poles (-68.6583, -135.7581) (-68.3523, -135.7792) (-67.8775, -135.7792) (-67.6031, -135.7581) knots 0 0 0 0 1 1 1 1
  spline S1530 degree 3 poles (-67.6031, -135.7581) (-67.3288, -135.737) (-67.582, -135.7264) (-68.1624, -135.7264) knots 0 0 0 0 1 1 1 1
  spline S1531 degree 3 poles (-68.1624, -135.7264) (-68.7427, -135.7264) (-68.9643, -135.737) (-68.6583, -135.7581) knots 0 0 0 0 1 1 1 1
  spline S1532 degree 3 poles (-43.9138, -135.7581) (-43.8189, -135.7792) (-43.65, -135.7792) (-43.5445, -135.7581) knots 0 0 0 0 1 1 1 1
  spline S1533 degree 3 poles (-43.5445, -135.7581) (-43.4495, -135.7264) (-43.5339, -135.7053) (-43.7344, -135.7053) knots 0 0 0 0 1 1 1 1
  spline S1534 degree 3 poles (-43.7344, -135.7053) (-43.9349, -135.7053) (-44.0193, -135.7264) (-43.9138, -135.7581) knots 0 0 0 0 1 1 1 1
  spline S1535 degree 3 poles (-43.0169, -135.7581) (-42.827, -135.7792) (-42.5421, -135.7792) (-42.3838, -135.7581) knots 0 0 0 0 1 1 1 1
  spline S1536 degree 3 poles (-42.3838, -135.7581) (-42.2255, -135.737) (-42.3838, -135.7159) (-42.732, -135.7159) knots 0 0 0 0 1 1 1 1
  spline S1537 degree 3 poles (-42.732, -135.7159) (-43.0802, -135.7159) (-43.2068, -135.737) (-43.0169, -135.7581) knots 0 0 0 0 1 1 1 1
  spline S1538 degree 3 poles (-42.9114, -136.5811) (-42.8903, -136.7289) (-42.8481, -136.8449) (-42.827, -136.8449) knots 0 0 0 0 1 1 1 1
  spline S1539 degree 3 poles (-42.827, -136.8449) (-42.8059, -136.8449) (-42.7848, -136.7289) (-42.7848, -136.5811) knots 0 0 0 0 1 1 1 1
  spline S1540 degree 3 poles (-42.7848, -136.5811) (-42.7848, -136.4334) (-42.827, -136.3173) (-42.8797, -136.3173) knots 0 0 0 0 1 1 1 1
  spline S1541 degree 3 poles (-42.8797, -136.3173) (-42.9219, -136.3173) (-42.943, -136.4334) (-42.9114, -136.5811) knots 0 0 0 0 1 1 1 1
  spline S1542 degree 3 poles (-42.521, -136.4123) (-42.6159, -136.4967) (-42.5737, -136.8449) (-42.4787, -136.8449) knots 0 0 0 0 1 1 1 1
  spline S1543 degree 3 poles (-42.4787, -136.8449) (-42.426, -136.8449) (-42.3943, -136.7711) (-42.4049, -136.6761) knots 0 0 0 0 1 1 1 1
  spline S1544 degree 3 poles (-42.4049, -136.6761) (-42.4049, -136.5811) (-42.331, -136.4862) (-42.2255, -136.4756) knots 0 0 0 0 1 1 1 1
  spline S1545 degree 3 poles (-42.2255, -136.4756) (-41.9511, -136.4228) (-41.9933, -136.8344) (-42.2783, -136.9504) knots 0 0 0 0 1 1 1 1
  spline S1546 degree 3 poles (-42.2783, -136.9504) (-42.4154, -137.0032) (-42.4682, -137.0454) (-42.4049, -137.0454) knots 0 0 0 0 1 1 1 1
  spline S1547 degree 3 poles (-42.4049, -137.0454) (-42.2044, -137.0665) (-41.4341, -136.6444) (-41.3813, -136.4756) knots 0 0 0 0 1 1 1 1
  spline S1548 degree 3 poles (-41.3813, -136.4756) (-41.3391, -136.3912) (-41.3602, -136.3173) (-41.413, -136.3173) knots 0 0 0 0 1 1 1 1
  spline S1549 degree 3 poles (-41.413, -136.3173) (-41.4763, -136.3173) (-41.5185, -136.3806) (-41.5185, -136.4651) knots 0 0 0 0 1 1 1 1
  spline S1550 degree 3 poles (-41.5185, -136.4651) (-41.5185, -136.5389) (-41.6135, -136.6339) (-41.7295, -136.6655) knots 0 0 0 0 1 1 1 1
  spline S1551 degree 3 poles (-41.7295, -136.6655) (-41.8667, -136.6972) (-41.9406, -136.6655) (-41.9406, -136.5811) knots 0 0 0 0 1 1 1 1
  spline S1552 degree 3 poles (-41.9406, -136.5811) (-41.9406, -136.4967) (-41.8562, -136.4228) (-41.7507, -136.3912) knots 0 0 0 0 1 1 1 1
  spline S1553 degree 3 poles (-41.7507, -136.3912) (-41.6557, -136.3701) (-41.7718, -136.349) (-42.025, -136.3595) knots 0 0 0 0 1 1 1 1
  spline S1554 degree 3 poles (-42.025, -136.3595) (-42.2677, -136.3595) (-42.4998, -136.3806) (-42.521, -136.4123) knots 0 0 0 0 1 1 1 1
  spline S1555 degree 3 poles (-41.1808, -136.5811) (-41.1808, -136.75) (-41.1597, -136.8133) (-41.1281, -136.7078) knots 0 0 0 0 1 1 1 1
  spline S1556 degree 3 poles (-41.1281, -136.7078) (-41.107, -136.6128) (-41.107, -136.4651) (-41.1281, -136.3912) knots 0 0 0 0 1 1 1 1
  spline S1557 degree 3 poles (-41.1281, -136.3912) (-41.1597, -136.3279) (-41.1808, -136.4017) (-41.1808, -136.5811) knots 0 0 0 0 1 1 1 1
  spline S1558 degree 3 poles (-44.1565, -136.7394) (-44.1565, -136.8555) (-44.2093, -136.9504) (-44.2726, -136.9504) knots 0 0 0 0 1 1 1 1
  spline S1559 degree 3 poles (-44.2726, -136.9504) (-44.3253, -136.9504) (-44.3465, -136.8977) (-44.3148, -136.8449) knots 0 0 0 0 1 1 1 1
  spline S1560 degree 3 poles (-44.3148, -136.8449) (-44.2831, -136.7816) (-44.3042, -136.7394) (-44.357, -136.7394) knots 0 0 0 0 1 1 1 1
  spline S1561 degree 3 poles (-44.357, -136.7394) (-44.4203, -136.7394) (-44.4731, -136.8133) (-44.4731, -136.8977) knots 0 0 0 0 1 1 1 1
  spline S1562 degree 3 poles (-44.4731, -136.8977) (-44.4731, -136.9821) (-44.3781, -137.056) (-44.262, -137.056) knots 0 0 0 0 1 1 1 1
  spline S1563 degree 3 poles (-44.262, -137.056) (-44.1038, -137.056) (-44.051, -136.9821) (-44.051, -136.7922) knots 0 0 0 0 1 1 1 1
  spline S1564 degree 3 poles (-44.051, -136.7922) (-44.051, -136.6444) (-44.0721, -136.5284) (-44.1038, -136.5284) knots 0 0 0 0 1 1 1 1
  spline S1565 degree 3 poles (-44.1038, -136.5284) (-44.1354, -136.5284) (-44.1565, -136.6233) (-44.1565, -136.7394) knots 0 0 0 0 1 1 1 1
  spline S1566 degree 3 poles (-43.8822, -136.6022) (-43.9138, -136.6444) (-43.9455, -136.7183) (-43.9455, -136.7816) knots 0 0 0 0 1 1 1 1
  spline S1567 degree 3 poles (-43.9455, -136.7816) (-43.9455, -136.8449) (-43.8927, -136.8238) (-43.84, -136.7394) knots 0 0 0 0 1 1 1 1
  spline S1568 degree 3 poles (-43.84, -136.7394) (-43.7555, -136.6128) (-43.7028, -136.6022) (-43.5234, -136.7078) knots 0 0 0 0 1 1 1 1
  spline S1569 degree 3 poles (-43.5234, -136.7078) (-43.2701, -136.866) (-42.9958, -136.8871) (-42.9958, -136.7394) knots 0 0 0 0 1 1 1 1
  spline S1570 degree 3 poles (-42.9958, -136.7394) (-42.9958, -136.6866) (-43.0697, -136.6761) (-43.1752, -136.7078) knots 0 0 0 0 1 1 1 1
  spline S1571 degree 3 poles (-43.1752, -136.7078) (-43.2807, -136.75) (-43.3229, -136.7289) (-43.2807, -136.6655) knots 0 0 0 0 1 1 1 1
  spline S1572 degree 3 poles (-43.2807, -136.6655) (-43.2068, -136.5495) (-43.7766, -136.4967) (-43.8822, -136.6022) knots 0 0 0 0 1 1 1 1
  spline S1573 degree 3 poles (-43.8611, -137.0243) (-43.7977, -137.0454) (-43.6711, -137.0454) (-43.5973, -137.0243) knots 0 0 0 0 1 1 1 1
  spline S1574 degree 3 poles (-43.5973, -137.0243) (-43.5339, -136.9927) (-43.5867, -136.9716) (-43.7344, -136.9716) knots 0 0 0 0 1 1 1 1
  spline S1575 degree 3 poles (-43.7344, -136.9716) (-43.8822, -136.9716) (-43.9349, -136.9927) (-43.8611, -137.0243) knots 0 0 0 0 1 1 1 1
  spline S1576 degree 3 poles (-43.3335, -137.0243) (-43.2596, -137.056) (-43.1646, -137.0454) (-43.133, -137.0138) knots 0 0 0 0 1 1 1 1
  spline S1577 degree 3 poles (-43.133, -137.0138) (-43.0908, -136.9821) (-43.1541, -136.9504) (-43.2701, -136.961) knots 0 0 0 0 1 1 1 1
  spline S1578 degree 3 poles (-43.2701, -136.961) (-43.3862, -136.961) (-43.4179, -136.9927) (-43.3335, -137.0243) knots 0 0 0 0 1 1 1 1
  spline S1579 degree 3 poles (-42.9114, -137.0243) (-42.8481, -137.0454) (-42.7214, -137.0454) (-42.6476, -137.0243) knots 0 0 0 0 1 1 1 1
  spline S1580 degree 3 poles (-42.6476, -137.0243) (-42.5843, -136.9927) (-42.637, -136.9716) (-42.7848, -136.9716) knots 0 0 0 0 1 1 1 1
  spline S1581 degree 3 poles (-42.7848, -136.9716) (-42.9325, -136.9716) (-42.9852, -136.9927) (-42.9114, -137.0243) knots 0 0 0 0 1 1 1 1
  spline S1582 degree 3 poles (-41.6979, -137.0243) (-41.5396, -137.0454) (-41.3075, -137.0454) (-41.1703, -137.0243) knots 0 0 0 0 1 1 1 1
  spline S1583 degree 3 poles (-41.1703, -137.0243) (-41.0437, -137.0032) (-41.1703, -136.9821) (-41.4657, -136.9821) knots 0 0 0 0 1 1 1 1
  spline S1584 degree 3 poles (-41.4657, -136.9821) (-41.7507, -136.9821) (-41.8667, -137.0032) (-41.6979, -137.0243) knots 0 0 0 0 1 1 1 1
extrude "Extrude4" cut sketch "Sketch6" against normal blind 0.2 contours S0 L4 L5 S1 L6 L7 S2 S3 S4 S5 S6 S7 S8 S9 S10 S11 S12 S13 S14 S15 S16 L8 L9 S17 S18 S19 S20 S21 S22 S23 S24 S25 S26 S27 S28 S29 S30 S31 S32 S33 S34 S35 S36 S37 L10 L11 S38 S39 S40 L12 L13 S41 S42 L14 L15 S43 S44 S45 S46 S47 S48 S49 S50 S51 S52 S53 S54 S55 S56 S57 S58 S59 S60 S61 S62 S63 S64 S65 S66 S67 S68 S69 S70 S71 S72 S73 S74 S75 L16 L17 L18 L19 S76 S77 S78 S79 S80 S81 S82 S83 S84 L20 L21 S85 S86 S87 L22 L23 L24 L25 S88 S89 S90 S91 S92 S93 S94 S95 S96 S97 S98 S99 S100 S101 S102 S103 S104 L26 L27 S105 S106 S107 S108 S109 S110 S111 S112 L28 L29 S113 S114 S115 S116 L30 L31 S117 S118 S119 S120 S121 S122 S123 S124 S125 S126 S127 L32 L33 S128 S129 S130 S131 S132 S133 S134 S135 S136 S137 S138 S139 S140 S141 S142 S143 S144 S145 S146 S147 S148 S149 S150 S151 S152 S153 S154 S155 S156 S157 S158 S159 S160 S161 S162 S163 S164 S165 S166 S167 S168 S169 S170 S171 S172 S173 S174 S175 S176 S177 S178 S179 L34 L35 S180 S181 S182 S183 S184 S185 S186 S187 S188 S189 S190 S191 L36 L37 S192 S193 S194 S195 S196 S197 S198 S199 S200 L38 L39 S201 S202 S203 S204 | S205 S206 S207 S208 L40 L41 S209 | S210 L42 L43 S211 S212 S213 S214 S215 S216 S217 S218 S219 S220 S221 S222 L44 L45 S223 S224 S225 S226 S227 S228 S229 S230 L46 L47 S231 S232 L48 L49 S233 S234 S235 L50 L51 S236 L52 L53 S237 S238 | S239 S240 L54 L55 S241 L56 L57 S242 S243 L58 L59 S244 S245 S246 S247 S248 S249 S250 S251 S252 S253 S254 L60 L61 S255 S256 S257 S258 S259 S260 S261 S262 S263 S264 S265 S266 S267 S268 S269 S270 S271 S272 S273 S274 S275 S276 S277 S278 S279 S280 S281 S282 S283 S284 S285 S286 | L62 L63 L64 L65 S287 S288 S289 S290 S291 S292 S293 | S294 S295 S296 S297 S298 | S299 S300 S301 S302 S303 | S304 S305 S306 S307 S308 S309 | S310 S311 S312 S313 S314 S315 S316 S317 | S318 L66 L67 S319 S320 S321 S322 S323 S324 S325 S326 S327 S328 S329 | S330 S331 S332 S333 S334 S335 S336 S337 S338 | S339 S340 S341 | L68 L69 S342 S343 S344 S345 L70 L71 S346 S347 | S348 S349 S350 S351 | S352 S353 S354 S355 S356 | S357 S358 S359 S360 L72 L73 L74 L75 S361 | S362 S363 S364 S365 S366 | S367 S368 S369 | S370 S371 S372 | S373 S374 S375 S376 S377 | S378 S379 S380 S381 S382 | S383 S384 S385 S386 S387 | S388 S389 S390 S391 S392 | S664 S665 L120 L121 L122 L123 S666 | S667 L124 L125 S668 S669 S670 S671 | S672 S673 S674 S675 L126 L127 S676 | S677 S678 S679 S680 S681 S682 S683 S684 S685 S686 S687 S688 S689 S690 S691 S692 S693 S694 S695 S696 S697 S698 S699 S700 S701 S702 L128 L129 S703 S704 S705 S706 S707 S708 S709 S710 S711 S712 S713 S714 S715 S716 L130 L131 S717 S718 S719 S720 S721 S722 S723 S724 S725 S726 S727 S728 S729 S730 S731 S732 S733 S734 S735 S736 S737 S738 S739 S740 L132 L133 S741 S742 S743 S744 S745 S746 S747 S748 S749 S750 S751 S752 S753 S754 S755 S756 S757 S758 S759 S760 | S761 S762 L134 L135 S763 S764 S765 L136 L137 S766 S767 | S768 S769 S770 | S771 S772 S773 S774 S775 S776 | S777 S778 S779 S780 S781 S782 S783 | S784 S785 S786 S787 | S788 S789 S790 S791 | S792 S793 S794 S795 | S796 S797 S798 | S799 S800 S801 S802 S803 L138 L139 S804 S805 S806 L140 L141 S807 S808 S809 | S810 S811 S812 S813 S814 S815 S816 | S817 L142 L143 S818 L144 L145 S819 S820 S821 | S822 S823 S824 S825 L146 L147 S826 S827 | S828 S829 S830 S831 S832 S833 L148 L149 S834 S835 | S836 S837 S838 S839 S840 S841 S842 | L150 L151 S843 S844 L152 L153 S845 S846 | S847 S848 S849 L154 L155 L156 L157 S850 | S851 L158 L159 S852 S853 | S854 S855 S856 S857 S858 S859 S860 S861 S862 | S863 L160 L161 S864 S865 S866 S867 L162 L163 L164 L165 S868 S869 S870 S871 S872 S873 S874 S875 S876 L166 L167 S877 S878 S879 S880 S881 S882 S883 S884 S885 S886 S887 | S888 S889 S890 S891 | S892 S893 S894 S895 S896 S897 S898 S899 | S900 S901 S902 S903 S904 S905 S906 S907 S908 S909 S910 S911 S912 | S913 S914 S915 S916 S917 S918 S919 S920 S921 S922 L168 L169 S923 S924 S925 S926 S927 S928 S929 S930 | S931 S932 S933 | S934 S935 S936 | S937 S938 S939 S940 | S941 S942 S943 S944 S945 S946 S947 | S948 S949 S950 S951 S952 | S953 S954 S955 | S956 S957 S958 S959 | S960 S961 S962 S963 S964 S965 S966 S967 S968 | S969 S970 S971 S972 S973 S974 | S975 S976 S977 S978 S979 S980 S981 | S982 L170 L171 S983 S984 S985 L172 L173 S986 S987 S988 S989 S990 S991 S992 S993 S994 S995 S996 S997 S998 S999 S1000 S1001 S1002 L174 L175 S1003 S1004 S1005 S1006 S1007 | S1008 S1009 S1010 | S1011 S1012 S1013 S1014 S1015 S1016 S1017 S1018 S1019 S1020 | S1021 S1022 S1023 S1024 S1025 S1026 S1027 S1028 S1029 S1030 | S1031 S1032 S1033 S1034 S1035 S1036 S1037 | S1038 S1039 S1040 | S1041 S1042 S1043 S1044 | S1045 S1046 S1047 S1048 | S1049 S1050 S1051 | S1052 S1053 S1054 S1055 | S1056 S1057 S1058 S1059 S1060 | S1061 S1062 S1063 S1064 | S1065 S1066 S1067 S1068 S1069 S1070 S1071 | S1072 S1073 S1074 S1075 | S1076 S1077 S1078 S1079 | S1080 S1081 S1082 S1083 S1084 S1085 | S1086 S1087 S1088 | S1089 S1090 S1091 S1092 | S1093 S1094 S1095 S1096 | S1097 S1098 S1099 S1100 S1101 S1102 S1103 S1104 S1105 S1106 S1107 S1108 S1109 S1110 L176 L177 S1111 S1112 S1113 | S1114 S1115 S1116 S1117 S1118 | S1119 S1120 S1121 L178 L179 | S1122 S1123 S1124 S1125 S1126 S1127 S1128 | S1129 S1130 S1131 | S1132 S1133 S1134 S1135 | S1136 S1137 S1138 S1139 | S1140 S1141 S1142 S1143 S1144 S1145 S1146 S1147 S1148 S1149 S1150 S1151 S1152 L180 L181 S1153 S1154 S1155 S1156 S1157 S1158 | S1159 S1160 S1161 | S1162 S1163 S1164 | S1165 S1166 S1167 S1168 | S1169 S1170 S1171 | S1172 S1173 S1174 S1175 | S1176 S1177 S1178 | S1179 S1180 S1181 S1182 | S1183 S1184 S1185 | S1186 S1187 L182 L183 S1188 S1189 S1190 S1191 S1192 S1193 S1194 S1195 | S1196 L184 L185 S1197 S1198 | S1199 S1200 S1201 | S1202 S1203 S1204 S1205 S1206 S1207 S1208 S1209 S1210 S1211 S1212 S1213 S1214 | S1215 L186 L187 S1216 S1217 | S1218 S1219 S1220 | S1221 S1222 S1223 S1224 S1225 S1226 S1227 S1228 S1229 S1230 S1231 S1232 S1233 S1234 | S1235 L188 L189 S1236 S1237 | S1238 S1239 S1240 | S1241 S1242 S1243 | S1244 S1245 S1246 S1247 S1248 S1249 S1250 | S1251 S1252 S1253 | S1254 S1255 S1256 S1257 | S1258 S1259 S1260 | S1261 S1262 S1263 S1264 S1265 S1266 S1267 | S1268 L190 L191 S1269 S1270 S1271 S1272 S1273 S1274 S1275 S1276 S1277 S1278 S1279 S1280 | S1281 S1282 S1283 | S1284 S1285 S1286 S1287 S1288 | S1289 S1290 S1291 S1292 | S1293 S1294 S1295 | S1296 S1297 S1298 | S1299 S1300 S1301 S1302 | S1303 S1304 S1305 | S1306 S1307 S1308 | S1309 S1310 S1311 S1312 S1313 | S1314 S1315 S1316 S1317 | S1318 S1319 S1320 | S1321 S1322 S1323 S1324 S1325 S1326 | S1327 S1328 S1329 S1330 S1331 S1332 S1333 S1334 S1335 S1336 S1337 S1338 S1339 S1340 S1341 S1342 S1343 | S1344 S1345 S1346 S1347 S1348 S1349 S1350 S1351 S1352 S1353 S1354 S1355 S1356 L192 L193 S1357 S1358 S1359 S1360 | S1361 S1362 S1363 | S1364 S1365 S1366 | S1367 S1368 S1369 S1370 S1371 S1372 | S1373 S1374 S1375 S1376 S1377 | S1378 S1379 S1380 | S1381 S1382 S1383 S1384 | S1385 S1386 S1387 S1388 S1389 S1390 S1391 S1392 S1393 S1394 S1395 | S1396 S1397 S1398 S1399 | S1400 S1401 S1402 S1403 S1404 S1405 S1406 S1407 S1408 S1409 | S1410 S1411 S1412 | S1413 S1414 S1415 S1416 | S1439 S1440 S1441 S1442 S1443 S1444 S1445 S1446 S1447 S1448 S1449 | S1450 S1451 S1452 S1453 | S1454 S1455 S1456 S1457 S1458 L196 L197 L198 L199 S1459 S1460 S1461 L200 L201 L202 L203 S1462 S1463 S1464 S1465 S1466 S1467 S1468 S1469 S1470 S1471 S1472 S1473 | S1474 S1475 S1476 S1477 S1478 | S1479 S1480 S1481 | S1482 S1483 S1484 | S1485 S1486 S1487 | S1488 S1489 S1490 S1491 S1492 S1493 S1494 S1495 S1496 S1497 S1498 S1499 L204 L205 S1500 L206 L207 S1501 S1502 | S1513 S1514 S1515 S1516 | S1517 S1518 S1519 S1520 | S1521 S1522 S1523 S1524 | S1525 S1526 S1527 S1528 | S1532 S1533 S1534 | S1535 S1536 S1537 | S1538 S1539 S1540 S1541 | S1542 S1543 S1544 S1545 S1546 S1547 S1548 S1549 S1550 S1551 S1552 S1553 S1554 | S1555 S1556 S1557 | S1558 S1559 S1560 S1561 S1562 S1563 S1564 S1565 | S1566 S1567 S1568 S1569 S1570 S1571 S1572 | S1573 S1574 S1575 | S1576 S1577 S1578 | S1579 S1580 S1581 | S1582 S1583 S1584 bodies 1
